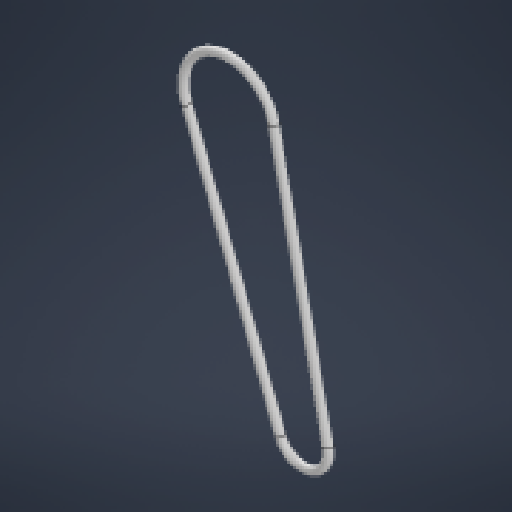
# Autodesk Inventor part: Belt
Saved by Autodesk Inventor 2024.2 (Build 282272000, 272)
## iProperties
Created: 2024-02-26
Part Number: Belt
Material: 一般
Document SubType Name: Modeling
Designer: Hanaoka
Density: 1 g/cm^3
Appearance: 既定
Author: Hanaoka
Autodesk Inventor part; units mm, degrees
ref_plane "YZ Plane" through (0, 0, 0) normal (1, 0, 0) x (0, 1, 0)
ref_plane "XZ Plane" through (0, 0, 0) normal (0, 1, 0) x (-1, 0, 0)
ref_plane "XY Plane" through (0, 0, 0) normal (0, 0, 1) x (1, 0, 0)
sketch "スケッチ1" plane through (0, 0, 0) normal (0, 0, 1) x (1, 0, 0)
  circle A0 centre (2, -12.5) radius 2.5 projected
  circle A1 centre (-7, 17.5) radius 5 projected
  line L0 (-2.1115, 18.5499) -> (4.4443, -11.9751)
  line L1 (-0.3296, -13.4072) -> (-11.6592, 15.6856)
  arc A2 (-1.1338, 18.7599) -> (-12.591, 15.3227) centre (-7, 17.5) ccw
  arc A3 (-1.2614, -13.7701) -> (5.422, -11.7651) centre (2, -12.5) ccw
  line L2 (-1.1338, 18.7599) -> (5.422, -11.7651)
  line L3 (-1.2614, -13.7701) -> (-12.591, 15.3227)
  point P0 (0, 0)
  dimension "d0" = 1
  dimension "d1" = 1
  constraints: 8 end point, 8 point on circle, 8 tangent, 2 centre point, 2 coincident
  measures "d0" radial gap between concentric circles of A1 A2
  measures "d1" radial gap between concentric circles of A3 A0
extrude "押し出し1" add sketch "スケッチ1" along normal blind 1
fillet "フィレット1" radius 0.5 16 edges at (2.7184, -14.8946, 1) (-5.9944, 1.1392, 1) (-8.4367, 22.2891, 1) (1.1664, 3.2874, 1) (-8.7241, 23.247, 1) (-6.9262, 0.7763, 1) (3.0057, -15.8524, 1) (2.1441, 3.4974, 1) (-8.7241, 23.247, 0) (-6.9262, 0.7763, 0) (3.0057, -15.8524, 0) (2.1441, 3.4974, 0) (2.7184, -14.8946, 0) (-5.9944, 1.1392, 0) (-8.4367, 22.2891, 0) (1.1664, 3.2874, 0)
